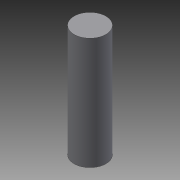
# Autodesk Inventor part: 18650
Saved by Autodesk Inventor 2015 (Build 190159000, 159)
## iProperties
Created: 2015-10-17
Part Number: 18650
Material: Generic
Document SubType Name: Modeling
Designer: Brian
Appearance: Default
Surface Area: 43.3281 cm^2
Volume: 17.5528 cm^3
Author: Brian
Autodesk Inventor part; units mm, degrees
ref_plane "YZ Plane" through (0, 0, 0) normal (1, 0, 0) x (0, 1, 0)
ref_plane "XZ Plane" through (0, 0, 0) normal (0, 1, 0) x (-1, 0, 0)
ref_plane "XY Plane" through (0, 0, 0) normal (0, 0, 1) x (1, 0, 0)
sketch "Sketch1" plane through (0, 0, 0) normal (0, 0, 1) x (1, 0, 0)
  circle A0 centre (0, 0) radius 9.25
  dimension "d0" = 18.5
  constraints: 1 centre point, 1 coincident
  measures "d0" diameter of A0
extrude "Extrusion1" add sketch "Sketch1" along normal blind 65.3
body "Solid1"
